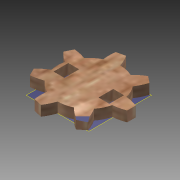
# Autodesk Inventor part: tandwiel(ja)
Saved by Autodesk Inventor 2015 (Build 190159000, 159)
## iProperties
Created: 2016-01-31
Part Number: tandwiel(ja)
Material: Generic
Document SubType Name: Modeling
Designer: david
Density: 1 g/cm^3
Appearance: Birch - Natural Polished
Author: david
Autodesk Inventor part; units mm, degrees
ref_plane "YZ Plane" through (0, 0, 0) normal (1, 0, 0) x (0, 1, 0)
ref_plane "XZ Plane" through (0, 0, 0) normal (0, 1, 0) x (-1, 0, 0)
ref_plane "XY Plane" through (0, 0, 0) normal (0, 0, 1) x (1, 0, 0)
ref_plane "Work Plane1" through (0, 0, 0) normal (0, 0, -1) x (-1, 0, 0)
sketch "Sketch3" plane through (0, 0, 0) normal (0, 0, -1) x (-1, 0, 0)
  circle A0 centre (0, 0) radius 11
  line L0 (-15.4, 0) -> (15.4, 0) projected
  dimension "d19" = 22
  constraints: 1 centre point, 1 coincident
  measures "d19" diameter of A0
extrude "Extrusion3" add sketch "Sketch3" against normal blind 3.6
sketch "Sketch4" plane through (0, 0, 3.6) normal (0, 0, 1) x (1, 0, 0)
  arc A0 (10.6524, -2.5) -> (10.6524, 2.5) centre (0, 0) ccw
  line L0 (-16.2075, 0) -> (20.2449, 0) projected
  line L1 (15, 0) -> (15, 1.5)
  arc A1 (15, 1.5) -> (10.6524, 2.5) centre (9.5012, -12.4558) ccw
  line L2 (15, 0) -> (15, -1.5)
  arc A2 (10.6524, -2.5) -> (15, -1.5) centre (9.5012, 12.4558) ccw
  dimension "d22" = 1.5
  dimension "d23" = 2.5
  dimension "d24" = 15
  dimension "d25" = 15
  constraints: 6 point on circle, 4 end point, 3 centre point, 3 symmetric about line, 1 coincident, 1 point on line, 1 vertical, 1 other
  measures "d22" distance of L1.start L1.end
  measures "d23" distance from line of L0 A0.end
  measures "d24" radius of A1
  measures "d25" distance from line of point (0, 0) L1
extrude "Extrusion4" add sketch "Sketch4" against normal blind 3.6
sketch "Sketch2" plane through (0, 0, 0) normal (0, 0, -1) x (-1, 0, 0)
  line L0 (-9.8, -2.6) -> (-6, -2.6)
  line L1 (-6, -2.6) -> (-6, 2.6)
  line L2 (-6, 2.6) -> (-9.8, 2.6)
  line L3 (-9.8, 2.6) -> (-9.8, -2.6)
  line L4 (-9.8, -2.6) -> (-6, 2.6) construction
  line L5 (-6, -2.6) -> (-9.8, 2.6) construction
  line L6 (0, -27.5637) -> (0, 32.5752)
  line L7 (9.8, -2.6) -> (6, -2.6)
  line L8 (6, -2.6) -> (6, 2.6)
  line L9 (6, 2.6) -> (9.8, 2.6)
  line L10 (9.8, 2.6) -> (9.8, -2.6)
  line L11 (9.8, -2.6) -> (6, 2.6) construction
  line L12 (6, -2.6) -> (9.8, 2.6) construction
  point P0 (-7.9, 0)
  point P1 (7.9, 0)
  point P2 (0, 0)
  dimension "d11" = 3.8
  dimension "d12" = 5.2
  dimension "d31" = 6
  dimension "d32" = 0
  constraints: 26 end point, 5 symmetric about line, 4 midpoint, 2 parallel, 1 horizontal, 1 perpendicular, 1 vertical
  measures "d11" distance of L2.end L1.end
  measures "d12" distance of L0.end L1.end
  measures "d31" distance from line of point (0, 0) L1
  measures "d32" distance from line of point (0, 0) L6
extrude "Extrusion2" cut sketch "Sketch2" against normal blind 3.6
pattern_circular "Circular Pattern1" count 7 over 360 about axis through (0, 0, 0) along (0, 0, 1) of "Extrusion4"
body "Solid1"
